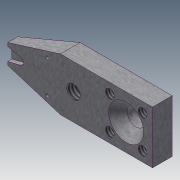
# Autodesk Inventor part: J005774
Saved by Autodesk Inventor 2015 SP1 (Build 190203100, 203)
## iProperties
Created: 2007-05-23
Document SubType Name: Modeling
Designer: komiyamat
Material: STAINLESS STEEL, 303
Density: 8 g/cm^3
Description: HEAD POST HOLDER BOTTOM
Appearance: Metal-Steel (Stainless, Brushed)
Part Number: J005774
Project: COMMON
Vendor: HHMI: JRC - ID&F
ALTERED ITEM DESCRIPTION: N/A
ALTERED ITEM PART NUMBER: N/A
ALTERED ITEM VENDOR: N/A
SPECIAL FINISH: NONE
SURFACE ROUGHNESS: 63 Ra
DESIGN DEPARTMENT: HHMI: JRC - ID&F
LAB/DEPT: COMMON
REQUESTING SCIENTIST: COMMON
Author: komiyamat
Revision Number: -
Autodesk Inventor part; units mm, degrees
ref_plane "YZ Plane" through (0, 0, 0) normal (1, 0, 0) x (0, 1, 0)
ref_plane "XZ Plane" through (0, 0, 0) normal (0, 1, 0) x (-1, 0, 0)
ref_plane "XY Plane" through (0, 0, 0) normal (0, 0, 1) x (1, 0, 0)
sketch "Sketch1" plane through (0, 0, 0) normal (0, 0, 1) x (1, 0, 0)
  line L0 (-25.4, 15.875) -> (-25.4, 3.175)
  line L1 (-25.4, 3.175) -> (9.525, 3.175)
  line L2 (9.525, 3.175) -> (9.525, 15.875)
  line L3 (9.525, 15.875) -> (-25.4, 15.875)
  dimension "d0" = 12.7
  dimension "d1" = 34.925
  constraints: 8 end point, 1 parallel, 1 vertical
  measures "d0" distance of L0.start L0.end
  measures "d1" distance of L0.end L1.end
extrude "Extrusion1" add sketch "Sketch1" along normal blind 4.7625
hole "Hole1" at (3.175, 9.525, 4.7625) direction (0, 0, -1) diameter 4.318 end through all countersink diameter 8.4328 countersink angle 82 clearance for "Flat Head Machine Screw (82)" size "#8" standard "Ansi Unified Screw Threads"
hole "Hole2" at (-9.525, 9.525, 4.7625) direction (0, 0, -1) diameter 3.302 end through all thread size "8-32 UNC" class "2B" standard "ANSI Unified Screw Threads"
sketch "Sketch2" plane through (0, 0, 4.7625) normal (0, 0, 1) x (1, 0, 0)
  line L0 (-25.4, 15.875) -> (9.525, 15.875) projected
  line L1 (-25.4, 3.175) -> (-25.4, 15.875) projected
  line L2 (-25.4, 11.1125) -> (-22.225, 11.1125)
  line L3 (-22.225, 11.1125) -> (-22.225, 7.9375)
  line L4 (-22.225, 7.9375) -> (-25.4, 7.9375)
  line L5 (-25.4, 7.9375) -> (-25.4, 11.1125)
  arc A0 (-22.225, 7.9375) -> (-22.225, 11.1125) centre (-22.225, 9.525) ccw
  dimension "d22" = 3.175
  dimension "d23" = 6.35
  dimension "d24" = 3.175
  constraints: 8 end point, 2 parallel, 2 point on circle, 2 tangent, 1 centre point, 1 horizontal, 1 perpendicular, 1 point on line
  measures "d22" distance of L3.end L4.end
  measures "d23" distance from line of L0 A0.centre
  measures "d24" distance between parallel lines of L4 L2
extrude "Extrusion2" cut sketch "Sketch2" against normal blind 1.016 contours L1 L2 L3 L4
sketch "Sketch6" plane through (-25.4, 3.175, 0) normal (0, -1, 0) x (1, 0, 0)
  line L0 (0, 0) -> (0, 4.7625) projected
  line L1 (0, 0) -> (34.925, 0) projected
  line L2 (0, 2.3813) -> (12.7, 0)
  line L3 (0, 0) -> (12.7, 0)
  line L4 (0, 0) -> (0, 2.3813)
  line L5 (0, 0) -> (12.7, 0)
  dimension "d35" = 2.3813
  dimension "d132" = 12.7
  constraints: 8 end point, 3 collinear, 1 midpoint, 1 point on line
  measures "d35" distance of L0.start L2.start
  measures "d132" distance of L0.start L2.end
extrude "Extrusion5" cut sketch "Sketch6" against normal through all
hole "Hole4" at (-15.875, 13.4938, 4.7625) direction (0, 0, -1) diameter 0.7874 end through all
hole "Hole6" at (-15.875, 5.5563, 4.7625) direction (0, 0, -1) diameter 0.7874 end through all
sketch "Sketch8" plane through (0, 0, 4.7625) normal (0, 0, 1) x (1, 0, 0)
  line L0 (-25.4, 11.1125) -> (-22.225, 11.1125) projected
  line L1 (-22.225, 11.1125) -> (-22.225, 7.9375) projected
  line L2 (-25.4, 11.1125) -> (-22.225, 11.1125)
  line L3 (-22.225, 10.3187) -> (-25.4, 11.1125)
  line L4 (-22.225, 11.1125) -> (-22.225, 10.3187)
  line L5 (-22.225, 8.7312) -> (-25.4, 7.9375)
  line L6 (-22.225, 7.9375) -> (-22.225, 8.7312)
  dimension "d80" = 0.7937
  dimension "d81" = 0.7937
  constraints: 10 end point, 3 collinear, 2 point on line
  measures "d80" distance of L0.end L3.start
  measures "d81" distance of L1.end L5.start
extrude "Extrusion7" add sketch "Sketch8" against normal up to next
sketch "Sketch10" plane through (0, 0, 4.7625) normal (0, 0, 1) x (1, 0, 0)
  line L0 (-22.225, 10.3187) -> (-22.225, 7.9375) projected
  line L1 (-22.225, 7.9375) -> (-25.4, 7.9375) projected
  line L2 (-22.225, 8.7312) -> (-25.4, 7.9375)
  line L3 (-22.225, 7.9375) -> (-22.225, 8.7312)
  dimension "d85" = 0.7937
  constraints: 4 end point, 1 collinear, 1 point on line
  measures "d85" distance of L0.end L2.start
extrude "Extrusion8" add sketch "Sketch10" against normal up to next
sketch "Sketch12" plane through (0, 0, 4.7625) normal (0, 0, 1) x (1, 0, 0)
  line L0 (-25.4, 15.875) -> (9.525, 15.875) projected
  line L1 (-25.4, 11.1125) -> (-25.4, 15.875) projected
  line L2 (-22.225, 10.3187) -> (-22.225, 8.7312) projected
  line L3 (-25.4, 11.9062) -> (-12.7, 15.875)
  line L4 (-25.4, 15.875) -> (-25.4, 11.9062)
  dimension "d88" = 12.7
  dimension "d89" = 3.9688
  constraints: 4 end point, 2 point on line, 1 parallel
  measures "d88" horizontal distance of L3.start L3.end
  measures "d89" vertical distance of L3.start L3.end
extrude "Extrusion9" cut sketch "Sketch12" against normal through all
sketch "Sketch13" plane through (0, 0, 4.7625) normal (0, 0, 1) x (1, 0, 0)
  line L0 (-25.4, 3.175) -> (-25.4, 7.9375) projected
  line L1 (9.525, 3.175) -> (-25.4, 3.175) projected
  line L2 (-12.7, 15.875) -> (9.525, 15.875) projected
  line L3 (-12.7, 3.175) -> (-25.4, 3.175)
  line L4 (-25.4, 7.1437) -> (-12.7, 3.175)
  dimension "d92" = 12.7
  dimension "d93" = 3.9688
  constraints: 4 end point, 2 point on line, 1 parallel
  measures "d92" horizontal distance of L4.start L3.start
  measures "d93" vertical distance of L4.start L3.start
extrude "Extrusion10" cut sketch "Sketch13" against normal through all
hole "Hole7" at (-0.7937, 13.4938, 4.7625) direction (0, 0, -1) diameter 2.159 end through all
hole "Hole8" at (-0.7937, 5.5562, 4.7625) direction (0, 0, -1) diameter 2.159 end through all
hole "Hole9" at (7.1437, 13.4938, 4.7625) direction (0, 0, -1) diameter 2.159 end through all
hole "Hole10" at (7.1437, 5.5562, 4.7625) direction (0, 0, -1) diameter 2.159 end through all
sketch "Sketch14" plane through (0, 0, 4.7625) normal (0, 0, 1) x (1, 0, 0)
  line L0 (-25.4, 11.1125) -> (-22.225, 10.3187) projected
  line L1 (-22.225, 8.7312) -> (-25.4, 7.9375) projected
  arc A0 (-22.225, 8.7312) -> (-22.225, 10.3187) centre (-22.4234, 9.525) ccw
  line L2 (-22.225, 10.3187) -> (-22.225, 8.7312)
  line L3 (-22.225, 8.7312) -> (-22.225, 10.3187) projected
  point P0 (0, 0)
  constraints: 2 end point, 2 point on circle, 1 centre point, 1 collinear, 1 tangent
extrude "Extrusion11" cut sketch "Sketch14" against normal up to surface (1.016 mm away)
body "Solid1"
